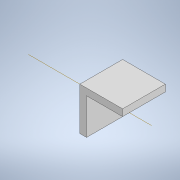
# Autodesk Inventor part: Angle Bracket
Saved by Autodesk Inventor 2022 (Build 260153000, 153)
## iProperties
Created: 2022-04-03
Part Number: Angle Bracket
Material: Generic
Document SubType Name: Modeling
Designer: Nick
Density: 1 g/cm^3
Appearance: Default
Author: Nick
Autodesk Inventor part; units mm, degrees
ref_plane "YZ Plane" through (0, 0, 0) normal (1, 0, 0) x (0, 1, 0)
ref_plane "XZ Plane" through (0, 0, 0) normal (0, 1, 0) x (-1, 0, 0)
ref_plane "XY Plane" through (0, 0, 0) normal (0, 0, 1) x (1, 0, 0)
sketch "Sketch1" plane through (0, 0, 0) normal (0, 0, 1) x (1, 0, 0)
  line L0 (0, 0) -> (0, 6.35)
  line L1 (0, 6.35) -> (6.35, 6.35)
  line L2 (6.35, 6.35) -> (6.35, 5.35)
  line L3 (6.35, 5.35) -> (1, 5.35)
  line L4 (1, 5.35) -> (1, 0)
  line L5 (1, 0) -> (0, 0)
  dimension "d0" = 6.35
  dimension "d1" = 6.35
  dimension "d2" = 1
  constraints: 12 end point, 2 horizontal, 2 perpendicular, 2 vertical, 1 parallel
  measures "d0" distance of L0.start L0.end
  measures "d1" distance of L0.end L1.end
  measures "d2" distance of L1.end L2.end
extrude "Extrusion1" add sketch "Sketch1" along normal blind 6.35
sketch "Sketch2" plane through (0, 0, 0) normal (-1, 0, 0) x (0, 0, 1)
  line L0 (6.35, 6.35) -> (6.35, 0) projected
  line L1 (0, 6.35) -> (6.35, 6.35) projected
  point P0 (0, 0)
  point P1 (3.175, 3.175)
  point P2 (6.35, 3.175)
  point P3 (3.175, 6.35)
  constraints: 2 midpoint, 1 horizontal alignment, 1 vertical alignment
equation "\"d1\" = d0"
body "Solid1"
